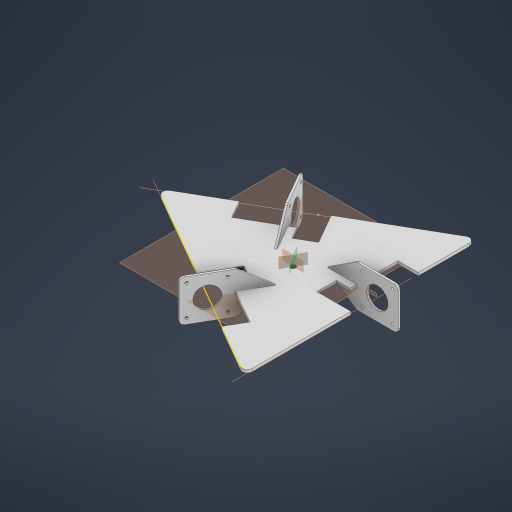
# Autodesk Inventor part: baseplate
Saved by Autodesk Inventor 2024 (Build 280153000, 153)
## iProperties
Created: 2026-03-23
Part Number: baseplate
Material: Generic
Document SubType Name: Modeling
Designer: schar
Density: 1 g/cm^3
Appearance: Default
Author: schar
Autodesk Inventor part; units mm, degrees
ref_plane "YZ Plane" through (0, 0, 0) normal (1, 0, 0) x (0, 1, 0)
ref_plane "XZ Plane" through (0, 0, 0) normal (0, 1, 0) x (-1, 0, 0)
ref_plane "XY Plane" through (0, 0, 0) normal (0, 0, 1) x (1, 0, 0)
sketch "Sketch1" plane through (0, 0, 0) normal (0, 1, 0) x (-1, 0, 0)
  line L0 (-61.782, 115.6699) -> (131.0641, 4.3301)
  line L1 (131.0641, -4.3301) -> (-61.782, -115.6699)
  line L2 (-69.282, -111.3397) -> (-69.282, 111.3397)
  arc A0 (131.0641, -4.3301) -> (131.0641, 4.3301) centre (128.5641, 0) ccw
  arc A1 (-69.282, -111.3397) -> (-61.782, -115.6699) centre (-64.282, -111.3397) ccw
  arc A2 (-61.782, 115.6699) -> (-69.282, 111.3397) centre (-64.282, 111.3397) ccw
  line L3 (34.641, -60) -> (-45.6615, 79.088)
  line L4 (-69.282, 0) -> (190.0751, 0)
  line L5 (34.641, 60) -> (-41.8401, -72.4692)
  circle A3 centre (0, 0) radius 2.5
  point P0 (0, 0)
  point P1 (-69.282, 120)
  point P2 (-69.282, -120)
  dimension "d5" = 240
  dimension "d9" = 60
  dimension "d10" = 60
  dimension "d14" = 5
  dimension "d25" = 5
  constraints: 12 end point, 6 point on circle, 6 point on line, 6 tangent, 4 centre point, 3 midpoint, 3 perpendicular, 2 equal radius, 1 coincident
  measures "d5" distance of point (-69.282, -120) point (-69.282, 120)
  measures "d9" angle of L1 L0
  measures "d10" angle of L1 L2
  measures "d14" radius of A0
  measures "d25" diameter of A3
extrude "Extrusion1" add sketch "Sketch1" along normal blind 3
sketch "Sketch2" plane through (0, 3, 0) normal (0, 1, 0) x (1, 0, 0)
  point P0 (0, 0)
ref_plane "Work Plane1" through (0, 1.5, 0) normal (0, 1, 0) x (1, 0, 0)
ref_plane "Work Plane2" through (0, 3, 0) normal (0.8660254, 0, 0.5) x (0, 1, 0)
ref_plane "Work Plane3" through (0, 3, 0) normal (-0.8660254, 0, 0.5) x (0, -1, 0)
ref_plane "Work Plane4" through (0, 3, 0) normal (0, 0, 1) x (1, 0, 0)
sketch "Sketch4" plane through (0, 3, 0) normal (0, 1, 0) x (1, 0, 0)
  point P0 (0, 0)
ref_plane "Work Plane5" through (0, 1.5, 0) normal (0, 1, 0) x (1, 0, 0)
ref_plane "Work Plane6" through (51.6025, 3, -19) normal (0, 0, 1) x (1, 0, 0)
sketch "Sketch6" plane through (0, 3, 0) normal (0, 1, 0) x (1, 0, 0)
  point P0 (0, 0)
sketch "Sketch7" plane through (0, 1.5, 0) normal (0, 1, 0) x (1, 0, 0)
  line L0 (-16.8875, -70.25) -> (-16.8875, -70.25)
  line L1 (-16.8875, -70.25) -> (-16.8875, -70.25)
  line L2 (-25.9808, -65) -> (-18.1865, -69.5)
  line L3 (-14.8875, -66.7859) -> (-16.8875, -70.25)
  line L4 (-14.1375, -65.4869) -> (-19.6375, -75.0131)
  line L5 (-19.6375, -75.0131) -> (-37.824, -64.5131)
  line L6 (-32.324, -54.9869) -> (-19.6375, -75.0131) construction
  line L7 (-37.824, -64.5131) -> (-32.324, -54.9869)
  line L8 (-37.824, -64.5131) -> (-14.1375, -65.4869) construction
  line L9 (-32.324, -54.9869) -> (-14.1375, -65.4869)
  line L10 (-8.4808, -34.6891) -> (-43.4808, -95.3109)
  line L11 (-60.8013, -85.3109) -> (-8.4808, -34.6891) construction
  line L12 (-60.8013, -85.3109) -> (-25.8013, -24.6891)
  line L13 (-25.8013, -24.6891) -> (-43.4808, -95.3109) construction
  line L14 (-7.6865, -51.3135) -> (-15.4808, -46.8135)
  line L15 (-25.9808, -65) -> (-8.4808, -34.6891)
  line L16 (-25.8013, -24.6891) -> (-8.4808, -34.6891)
  line L17 (-16.8875, -70.25) -> (-14.8875, -66.7859)
  line L18 (-18.1865, -69.5) -> (-7.6865, -51.3135)
  line L19 (16.4545, -89.5) -> (-18.1865, -69.5)
  line L20 (-7.6865, -51.3135) -> (26.9545, -71.3135)
  line L21 (26.9545, -71.3135) -> (16.4545, -89.5)
  line L22 (-14.8875, -66.7859) -> (-14.8875, -66.7859)
  line L23 (-43.4808, -95.3109) -> (-60.8013, -85.3109)
  line L24 (-34.641, -60) -> (-25.9808, -65)
  line L25 (-131.0641, -4.3301) -> (61.782, -115.6699) projected
  line L26 (69.282, 20.5) -> (69.282, 20.5)
  line L27 (69.282, 20.5) -> (69.282, 20.5)
  line L28 (104.282, 10) -> (104.282, -10)
  line L29 (74.782, -0.5) -> (63.782, -0.5)
  line L30 (69.282, 0) -> (69.282, 10)
  line L31 (104.282, -10) -> (34.282, -10)
  line L32 (63.782, -0.5) -> (74.782, 20.5) construction
  line L33 (74.782, 20.5) -> (74.782, -0.5)
  line L34 (104.282, -10) -> (34.282, 10) construction
  line L35 (34.282, -10) -> (104.282, 10) construction
  line L36 (63.782, -0.5) -> (63.782, 20.5)
  line L37 (74.782, -0.5) -> (63.782, 20.5) construction
  line L38 (34.282, -10) -> (34.282, 10)
  line L39 (34.282, 10) -> (104.282, 10)
  line L40 (69.282, 10) -> (34.282, 10)
  line L41 (65.282, 20.5) -> (69.282, 20.5)
  line L42 (65.282, 20.5) -> (65.282, 20.5)
  line L43 (69.282, 20.5) -> (65.282, 20.5)
  line L44 (63.782, 20.5) -> (74.782, 20.5)
  line L45 (69.282, 19) -> (48.282, 19)
  line L46 (69.282, 59) -> (69.282, 19)
  line L47 (69.282, 10) -> (69.282, 19)
  line L48 (48.282, 59) -> (69.282, 59)
  line L49 (48.282, 19) -> (48.282, 10)
  line L50 (48.282, 19) -> (48.282, 59)
  line L51 (-52.3945, 49.75) -> (-52.3945, 49.75)
  line L52 (-52.3945, 49.75) -> (-52.3945, 49.75)
  line L53 (-60.8013, 85.3109) -> (-43.4808, 95.3109)
  line L54 (-36.958, 65.0131) -> (-31.458, 55.4869)
  line L55 (-34.641, 60) -> (-43.3013, 55)
  line L56 (-43.4808, 95.3109) -> (-8.4808, 34.6891)
  line L57 (-31.458, 55.4869) -> (-55.1445, 54.5131) construction
  line L58 (-55.1445, 54.5131) -> (-36.958, 65.0131)
  line L59 (-43.4808, 95.3109) -> (-25.8013, 24.6891) construction
  line L60 (-8.4808, 34.6891) -> (-60.8013, 85.3109) construction
  line L61 (-31.458, 55.4869) -> (-49.6445, 44.9869)
  line L62 (-36.958, 65.0131) -> (-49.6445, 44.9869) construction
  line L63 (-8.4808, 34.6891) -> (-25.8013, 24.6891)
  line L64 (-25.8013, 24.6891) -> (-60.8013, 85.3109)
  line L65 (-43.3013, 55) -> (-25.8013, 24.6891)
  line L66 (-50.3945, 46.2859) -> (-52.3945, 49.75)
  line L67 (-50.3945, 46.2859) -> (-50.3945, 46.2859)
  line L68 (-52.3945, 49.75) -> (-50.3945, 46.2859)
  line L69 (-49.6445, 44.9869) -> (-55.1445, 54.5131)
  line L70 (-51.0955, 50.5) -> (-40.5955, 32.3135)
  line L71 (-85.7365, 30.5) -> (-51.0955, 50.5)
  line L72 (-43.3013, 55) -> (-51.0955, 50.5)
  line L73 (-75.2365, 12.3135) -> (-85.7365, 30.5)
  line L74 (-40.5955, 32.3135) -> (-32.8013, 36.8135)
  line L75 (-40.5955, 32.3135) -> (-75.2365, 12.3135)
  point P0 (0, 0)
  point P1 (-34.641, -60)
  point P2 (-16.8875, -70.25)
  point P3 (-28.7308, -69.7631)
  point P4 (-34.641, -60)
  point P5 (0, 0)
  point P6 (69.282, 111.3397)
  point P7 (69.282, 0)
  point P8 (69.282, 0)
  point P9 (0, 0)
  point P10 (-131.0641, 4.3301)
  point P11 (-34.641, 60)
  point P12 (-34.641, 60)
  point P13 (69.282, 20.5)
  point P14 (74.782, 10)
  point P15 (-52.3945, 49.75)
  point P16 (-46.0513, 59.7631)
  dimension "d59" = 10
  dimension "d60" = 35
  dimension "d61" = 11
  dimension "d62" = 21
  dimension "d63" = 4
  dimension "d64" = 9
  dimension "d65" = 21
  dimension "d66" = 40
  dimension "d129" = 360
  constraints: 150 end point, 11 perpendicular, 10 midpoint, 8 parallel, 6 point on line, 2 coincident, 146 other
  measures "d59" distance of L24.start L2.start
  measures "d60" distance of L2.start L10.start
  measures "d61" distance of L8.start L6.start
  measures "d62" distance of L6.start L4.start
  measures "d63" distance of L22.end L1.start
  measures "d64" distance of L2.start L2.end
  measures "d65" distance of L2.end L18.end
  measures "d66" distance of L18.end L21.start
extrude "Extrusion3" cut sketch "Sketch7" along normal mid plane 3
sketch "Sketch9" plane through (0, 3, 0) normal (0, 1, 0) x (1, 0, 0)
  line L0 (-131.0641, -4.3301) -> (61.782, -115.6699) projected
  point P0 (0, 0)
  point P1 (-34.641, -60)
  constraints: 1 midpoint
ref_plane "Work Plane8" through (-0.6865, 0, 39.1891) normal (-0.8660254, 0, -0.5) x (-0.5, 0, 0.8660254)
sketch "Sketch13" plane through (0, 3, 0) normal (0, 1, 0) x (1, 0, 0)
  circle A0 centre (0, 0) radius 2.5
  dimension "d124" = 5
  constraints: 1 centre point, 1 coincident
  measures "d124" diameter of A0
extrude "Extrusion7" cut sketch "Sketch13" against normal through all
ref_plane "Work Plane9" through (-33.5955, 0, -20.1891) normal (0.8660254, 0, -0.5) x (-0.5, 0, -0.8660254)
sketch "Sketch14" plane through (51.6025, 3, -19) normal (0, 0, 1) x (1, 0, 0)
  line L0 (10.1795, 0) -> (-77.5833, 0) projected
  line L1 (-3.2665, 0) -> (-13.2665, 0)
  line L2 (10.1795, -3) -> (-77.5833, -3) projected
  line L3 (-13.2665, -3) -> (-3.2665, -3)
  line L4 (-3.3205, -3) -> (-3.3205, 0) projected
  line L5 (-3.3205, -1.5) -> (17.8295, -1.5)
  line L6 (38.9795, 19.65) -> (-3.3205, 19.65)
  line L7 (-3.3205, 19.65) -> (-3.3205, -22.65)
  line L8 (-3.3205, -22.65) -> (38.9795, -22.65)
  line L9 (38.9795, -22.65) -> (38.9795, 19.65)
  line L10 (38.9795, 19.65) -> (-3.3205, -22.65) construction
  line L11 (-3.3205, 19.65) -> (38.9795, -22.65) construction
  line L12 (2.3295, -17) -> (33.3295, -17)
  line L13 (33.3295, -17) -> (33.3295, 14)
  line L14 (33.3295, 14) -> (2.3295, 14)
  line L15 (2.3295, 14) -> (2.3295, -17)
  line L16 (2.3295, -17) -> (33.3295, 14) construction
  line L17 (33.3295, -17) -> (2.3295, 14) construction
  circle A0 centre (2.3295, 14) radius 1.5
  circle A1 centre (33.3295, 14) radius 1.5
  circle A2 centre (33.3295, -17) radius 1.5
  circle A3 centre (2.3295, -17) radius 1.5
  line L18 (-13.2665, 0) -> (-23.2665, 0)
  line L19 (-3.3205, 0) -> (-33.3205, 0)
  line L20 (-33.3205, 0) -> (-3.3205, 19.65)
  line L21 (-33.3205, -3) -> (-3.3205, -22.65)
  line L22 (-3.3205, -3) -> (2.3295, -3)
  line L23 (2.3295, -3) -> (2.3295, 0)
  line L24 (2.3295, 0) -> (-3.3205, 0)
  line L25 (-3.3205, 0) -> (-3.3205, -3)
  circle A4 centre (17.8295, -1.5) radius 11
  point P0 (-51.6025, -3)
  dimension "d133" = 21.15
  dimension "d134" = 42.3
  dimension "d135" = 31
  dimension "d136" = 31
  dimension "d137" = 3
  dimension "d138" = 3
  dimension "d139" = 3
  dimension "d140" = 3
  dimension "d142" = 30
  dimension "d145" = 22
  constraints: 46 end point, 9 point on line, 6 parallel, 5 centre point, 5 coincident, 5 midpoint, 4 perpendicular, 3 horizontal
  measures "d133" distance of L5.start L5.end
  measures "d134" distance of L7.end L6.end
  measures "d135" distance of L14.end L13.end
  measures "d136" distance of L13.end L12.end
  measures "d137" diameter of A0
  measures "d138" diameter of A1
  measures "d139" diameter of A2
  measures "d140" diameter of A3
  measures "d142" distance of L4.end L19.end
  measures "d145" diameter of A4
extrude "Extrusion8" add sketch "Sketch14" along normal blind 2 contours L15 L5 L4 L0 | L15 A0 L14 A1 L13 A2 L12 A3 L2 A4 L0 | L0 L7 L6 L9 L8 L2 L15 A3 L12 A2 L13 A1 L14 A0 | L0 A4 L5 L15 | L15 L2 L4 L5 | L5 A4 L2 L15 | L0 L20 L7 | L7 L21 L2
fillet "Fillet1" radius 4 4 edges at (90.582, 22.65, -18) (90.582, -19.65, -18) (48.282, 22.65, -18) (48.282, -19.65, -18)
pattern_circular "Circular Pattern1" count 3 over 360 about axis through (0, 3, 0) along (0, -1, 0) of "Extrusion8", "Fillet1"
body "Solid1"
